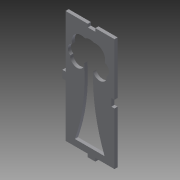
# Autodesk Inventor part: Birdhouse Wall 2
Saved by Autodesk Inventor 2015 (Build 190159000, 159)
## iProperties
Created: 2018-03-09
Part Number: Birdhouse Wall 2
Material: Generic
Document SubType Name: Modeling
Designer: Administrator
Density: 1 g/cm^3
Appearance: Default
Author: Administrator
Autodesk Inventor part; units mm, degrees
ref_plane "YZ Plane" through (0, 0, 0) normal (1, 0, 0) x (0, 1, 0)
ref_plane "XZ Plane" through (0, 0, 0) normal (0, 1, 0) x (-1, 0, 0)
ref_plane "XY Plane" through (0, 0, 0) normal (0, 0, 1) x (1, 0, 0)
sketch "Sketch1" plane through (0, 0, 0) normal (0, 0, 1) x (1, 0, 0)
  line L0 (0, 0) -> (49.7586, 0)
  line L1 (49.7586, 0) -> (49.7586, 114.3)
  line L2 (49.7586, 114.3) -> (0, 114.3)
  line L3 (0, 114.3) -> (0, 0)
  dimension "d0" = 114.3
  dimension "d1" = 49.7586
  constraints: 8 end point, 2 parallel, 1 horizontal, 1 perpendicular
  measures "d0" distance of L2.end L0.start
  measures "d1" distance of L0.start L0.end
extrude "Extrusion1" add sketch "Sketch1" along normal blind 3.175
sketch "Sketch2" plane through (0, 0, 3.175) normal (0, 0, 1) x (1, 0, 0)
  line L0 (0, 114.3) -> (0, 0) projected
  line L1 (49.7586, 0) -> (49.7586, 114.3) projected
  line L2 (0, 60.96) -> (-3.175, 60.96)
  line L3 (-3.175, 60.96) -> (-3.175, 53.34)
  line L4 (-3.175, 53.34) -> (0, 53.34)
  line L5 (0, 53.34) -> (0, 60.96)
  line L6 (49.7586, 60.96) -> (46.5836, 60.96)
  line L7 (46.5836, 60.96) -> (46.5836, 53.34)
  line L8 (46.5836, 53.34) -> (49.7586, 53.34)
  line L9 (49.7586, 53.34) -> (49.7586, 60.96)
  line L10 (49.7586, 114.3) -> (0, 114.3) projected
  line L11 (0, 0) -> (49.7586, 0) projected
  line L12 (30.2514, 114.3) -> (22.6314, 114.3)
  line L13 (30.2514, 0) -> (30.2514, -3.175)
  line L14 (30.2514, -3.175) -> (22.6314, -3.175)
  line L15 (22.6314, -3.175) -> (22.6314, 0)
  line L16 (22.6314, 0) -> (30.2514, 0)
  line L17 (22.6314, 114.3) -> (22.6314, 111.125)
  line L18 (22.6314, 111.125) -> (30.2514, 111.125)
  line L19 (30.2514, 111.125) -> (30.2514, 114.3)
  point P0 (0, 57.15)
  point P1 (49.7586, 57.15)
  point P2 (26.4414, 0)
  point P3 (26.4414, 114.3)
  dimension "d4" = 3.81
  dimension "d5" = 7.62
  dimension "d6" = 3.175
  dimension "d7" = 3.81
  dimension "d8" = 7.62
  dimension "d9" = 3.175
  dimension "d13" = 7.62
  dimension "d15" = 3.175
  dimension "d20" = 7.62
  dimension "d22" = 3.175
  dimension "d33" = 3.81
  dimension "d34" = 26.4414
  dimension "d35" = 26.4414
  dimension "d36" = 3.81
  constraints: 32 end point, 8 point on line, 7 perpendicular, 6 parallel, 4 midpoint, 2 collinear, 2 vertical
  measures "d4" distance from line of point (0, 57.15) L2
  measures "d5" distance between parallel lines of L2 L4
  measures "d6" distance between parallel lines of L0 L3
  measures "d7" distance from line of point (49.759, 57.15) L6
  measures "d8" distance between parallel lines of L6 L8
  measures "d9" distance between parallel lines of L1 L7
  measures "d13" distance between parallel lines of L13 L15
  measures "d15" distance between parallel lines of L14 L11
  measures "d20" distance between parallel lines of L17 L19
  measures "d22" distance between parallel lines of L10 L18
  measures "d33" distance from line of L13 point (26.441, 0)
  measures "d34" distance from line of point (26.441, 0) L0
  measures "d35" distance from line of L0 point (26.441, 114.3)
  measures "d36" distance from line of L19 point (26.441, 114.3)
extrude "Extrusion2" add sketch "Sketch2" against normal blind 3.175 contours L0 L4 L3 L2 | L10 L19 L18 L17 | L11 L13 L14 L15 | L1 L8 L7 L6
extrude "Extrusion3" cut sketch "Sketch2" against normal blind 3.175 contours L10 L19 L18 L17 | L1 L8 L7 L6
sketch "Sketch3" plane through (0, 0, 3.175) normal (0, 0, 1) x (1, 0, 0)
  line L0 (0, 60.96) -> (0, 114.3)
  line L1 (22.6314, 114.3) -> (0, 114.3) projected
  line L2 (0, 114.3) -> (22.6314, 114.3)
  line L3 (22.6314, 114.3) -> (22.6314, 111.125)
  line L4 (22.6314, 111.125) -> (30.2514, 111.125)
  line L5 (30.2514, 111.125) -> (22.6314, 111.125) projected
  line L6 (30.2514, 111.125) -> (30.2514, 114.3)
  line L7 (30.2514, 114.3) -> (49.7586, 114.3)
  line L8 (49.7586, 114.3) -> (49.7586, 60.96)
  line L9 (49.7586, 60.96) -> (49.7586, 114.3) projected
  line L10 (49.7586, 60.96) -> (46.5836, 60.96)
  line L11 (46.5836, 60.96) -> (46.5836, 53.34)
  line L12 (46.5836, 60.96) -> (46.5836, 53.34) projected
  line L13 (46.5836, 53.34) -> (49.7586, 53.34)
  line L14 (49.7586, 53.34) -> (49.7586, 0)
  line L15 (49.7586, 0) -> (49.7586, 53.34) projected
  line L16 (49.7586, 0) -> (30.2514, 0)
  line L17 (0, 0) -> (22.6314, 0) projected
  line L18 (30.2514, 0) -> (30.2514, -3.175)
  line L19 (30.2514, -3.175) -> (22.6314, -3.175)
  line L20 (22.6314, -3.175) -> (30.2514, -3.175) projected
  line L21 (22.6314, -3.175) -> (22.6314, 0)
  line L22 (22.6314, 0) -> (0, 0)
  line L23 (0, 0) -> (0, 53.34)
  line L24 (0, 53.34) -> (0, 0) projected
  line L25 (0, 53.34) -> (-3.175, 53.34)
  line L26 (-3.175, 53.34) -> (-3.175, 60.96)
  line L27 (-3.175, 60.96) -> (-3.175, 53.34) projected
  line L28 (-3.175, 60.96) -> (0, 60.96)
  constraints: 40 end point, 10 perpendicular, 9 collinear
sketch "Sketch4" plane through (0, 0, 3.175) normal (0, 0, 1) x (1, 0, 0)
  arc A0 (9.4645, 6.35) -> (18.9927, 77.7875) centre (-158.3531, 65.0875) ccw
  arc A1 (28.1243, 77.7875) -> (39.6875, 6.35) centre (205.7485, 69.884) ccw
  line L0 (0, 0) -> (22.6314, 0) projected
  line L1 (30.2514, 0) -> (49.7586, 0) projected
  line L2 (9.4645, 6.35) -> (39.6875, 6.35)
  arc A2 (4.7619, 76.2078) -> (18.9927, 77.7875) centre (11.8465, 77.2757) ccw
  arc A3 (6.7319, 88.6305) -> (4.6889, 77.5927) centre (8.7235, 82.5539) ccw
  arc A4 (4.6889, 77.5927) -> (4.7619, 76.2078) centre (11.8465, 77.2757) ccw
  arc A5 (19.9033, 100.0791) -> (6.7319, 88.6305) centre (15.9469, 91.3299) ccw
  line L3 (23.3172, 114.3) -> (23.3172, 47.625) construction
  line L4 (49.7586, 60.96) -> (49.7586, 114.3) projected
  arc A6 (28.02, 74.925) -> (41.8725, 76.2078) centre (34.7879, 77.2757) ccw
  arc A7 (41.9455, 77.5927) -> (39.9025, 88.6305) centre (37.9109, 82.5539) ccw
  arc A8 (41.8725, 76.2078) -> (41.9455, 77.5927) centre (34.7879, 77.2757) ccw
  arc A9 (39.9025, 88.6305) -> (28.7277, 100.7299) centre (30.6875, 91.3299) ccw
  arc A10 (28.7277, 100.7299) -> (19.9033, 100.0791) centre (24.8672, 92.9247) ccw
  point P0 (21.8385, 98.9122)
  point P1 (27.6417, 77.7875)
  point P2 (24.7959, 98.9122)
  dimension "d23" = 71.4375
  dimension "d24" = 6.35
  dimension "d25" = 177.8
  dimension "d26" = 6.35
  dimension "d28" = 177.8
  dimension "d29" = 26.4414
  dimension "d30" = 71.4375
  constraints: 23 point on circle, 11 centre point, 9 symmetric about line, 4 end point, 1 tangent, 1 vertical, 4 other
  measures "d23" vertical distance of L2.start A0.end
  measures "d24" distance from line of L0 L2.start
  measures "d25" radius of A0
  measures "d26" distance from line of L1 L2.end
  measures "d28" radius of A1
  measures "d29" distance between parallel lines of L4 L3
  measures "d30" vertical distance of A1.start L2.end
extrude "Extrusion4" cut sketch "Sketch4" against normal blind 25.4
body "Solid1"
